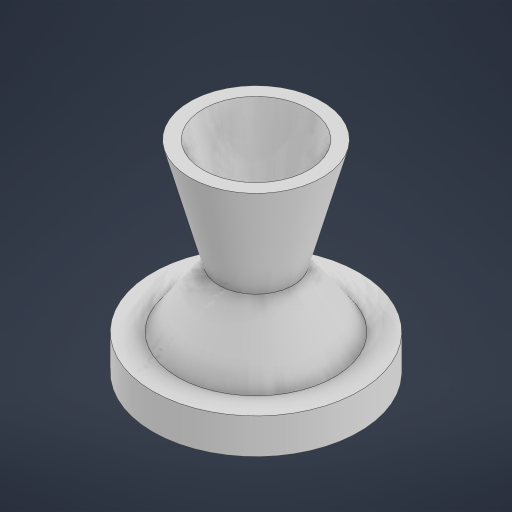
# Autodesk Inventor part: nozzle
Saved by Autodesk Inventor 2023 (Build 270158000, 158)
## iProperties
Created: 2022-10-07
Part Number: nozzle
Material: Generic
Document SubType Name: Modeling
Designer: washington
Density: 1 g/cm^3
Appearance: Default
Author: washington
Autodesk Inventor part; units mm, degrees
ref_plane "YZ Plane" through (0, 0, 0) normal (1, 0, 0) x (0, 1, 0)
ref_plane "XZ Plane" through (0, 0, 0) normal (0, 1, 0) x (-1, 0, 0)
ref_plane "XY Plane" through (0, 0, 0) normal (0, 0, 1) x (1, 0, 0)
sketch "Sketch1" plane through (0, 0, 0) normal (1, 0, 0) x (0, 1, 0)
  line L0 (0, 22.4) -> (23.4216, 6)
  line L1 (23.4216, 6) -> (45.8139, 12)
  line L2 (45.8139, 12) -> (45.8139, 15)
  line L3 (45.8139, 15) -> (21.3558, 8.4465)
  line L4 (21.3558, 8.4465) -> (8, 17.7983)
  line L5 (8, 17.7983) -> (8, 23.4)
  line L6 (8, 23.4) -> (0, 23.4)
  line L7 (0, 23.4) -> (0, 22.4)
  line L8 (-9.1628, 0) -> (54.9767, 0) projected
  point P0 (0, 0)
  dimension "d0" = 23.4
  dimension "d1" = 8
  dimension "d3" = 6
  dimension "d4" = 1
  dimension "d5" = 35
  dimension "d6" = 15
  dimension "d7" = 12
  dimension "d8" = 3
  dimension "d9" = 45.8139
  constraints: 16 end point, 3 parallel, 2 perpendicular, 1 point on line, 1 vertical
  measures "d0" distance from line of L6 point (0, 0)
  measures "d1" distance between parallel lines of L7 L5
  measures "d3" vertical distance of point (0, 0) L0.end
  measures "d4" distance of L6.end L0.start
  measures "d5" angle of L6 L0
  measures "d6" angle of L6 L1
  measures "d7" vertical distance of point (0, 0) L1.end
  measures "d8" distance of L1.end L2.end
  measures "d9" distance from line of point (0, 0) L2
revolve "Revolution1" add sketch "Sketch1" angle 360 about axis through (0, -10, 0) along (0, 1, 0)
body "Solid1"
